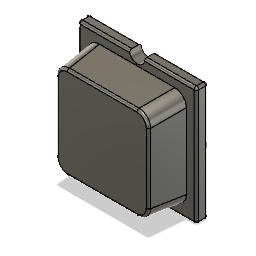
senseCam_Adapter_rev2_enclosure_V2 (Autodesk Fusion 360 archive; units mm, degrees)
design "CA16372_HB-SQ-WWW_Single_Lens"
Autodesk Fusion 360 part; units mm, degrees
sketch "Base 1" plane through (0, 0, 0) normal (0, 0, 1) x (1, 0, 0)
  line L0 (12.5, 12.5) -> (-12.5, 12.5)
  line L1 (-12.5, 12.5) -> (-12.5, -12.5)
  line L2 (-12.5, -12.5) -> (12.5, -12.5)
  line L3 (12.5, -12.5) -> (12.5, 12.5)
  line L4 (12.5, 12.5) -> (-12.5, -12.5) construction
  line L5 (-12.5, 12.5) -> (12.5, -12.5) construction
  line L6 (12.7, 12.7) -> (-12.7, 12.7)
  line L7 (-12.7, 12.7) -> (-12.7, -12.7)
  line L8 (-12.7, -12.7) -> (12.7, -12.7)
  line L9 (12.7, -12.7) -> (12.7, 12.7)
  line L10 (12.7, 12.7) -> (-12.7, -12.7) construction
  line L11 (-12.7, 12.7) -> (12.7, -12.7) construction
  circle A0 centre (0, 12.5) radius 1.6
  circle A1 centre (0, -12.5) radius 1.6
  dimension "d1" = 25
  dimension "d2" = 25
  dimension "d3" = 25.4
  dimension "d4" = 25.4
  dimension "d5" = 3.2
  dimension "d6" = 3.2
  constraint perpendicular L0 L1
  constraint parallel L0 L2
  constraint parallel L1 L3
  constraint horizontal L0
  constraint coincident L4 origin
  constraint coincident L5 origin
  constraint perpendicular L6 L7
  constraint parallel L6 L8
  constraint parallel L7 L9
  constraint horizontal L6
  constraint coincident L10 origin
  constraint coincident L11 origin
  constraint midpoint L0 A0.centre
  constraint midpoint L2 A1.centre
  measures "d1" distance of L0.end L1.end
  measures "d2" distance of L1.end L2.end
  measures "d3" distance of L7.end L8.end
  measures "d4" distance of L6.end L7.end
  measures "d5" diameter of A0
  measures "d6" diameter of A1
extrude "Extrude1" add sketch "Base 1" along normal blind 2.49 contours L0 L1 L2 L3 A0 A1 | L0 L2 L3 L6 L8 L9 A0 A1 | L0 L1 L2 L6 L7 L8 A0 A1
sketch "Lens 1" plane through (0, 0, 2.49) normal (0, 0, 1) x (1, 0, 0)
  line L0 (12.7, -12.7) -> (12.7, 12.7)
  line L1 (12.7, 12.7) -> (1.5875, 12.7)
  arc A0 (-1.5875, 12.7) -> (1.5875, 12.7) centre (0, 12.5) ccw
  line L2 (-1.5875, 12.7) -> (-12.7, 12.7)
  line L3 (-12.7, 12.7) -> (-12.7, -12.7)
  line L4 (-12.7, -12.7) -> (-1.5875, -12.7)
  arc A1 (1.5875, -12.7) -> (-1.5875, -12.7) centre (0, -12.5) ccw
  line L5 (1.5875, -12.7) -> (12.7, -12.7)
  line L6 (10.76, 10.76) -> (-10.76, 10.76)
  line L7 (-10.76, 10.76) -> (-10.76, -10.76)
  line L8 (-10.76, -10.76) -> (10.76, -10.76)
  line L9 (10.76, -10.76) -> (10.76, 10.76)
  line L10 (10.76, 10.76) -> (-10.76, -10.76) construction
  line L11 (-10.76, 10.76) -> (10.76, -10.76) construction
  dimension "d9" = 21.52
  dimension "d10" = 21.52
  constraint perpendicular L6 L7
  constraint parallel L6 L8
  constraint parallel L7 L9
  constraint horizontal L6
  constraint coincident L10 origin
  constraint coincident L11 origin
  measures "d9" distance of L7.end L8.end
  measures "d10" distance of L6.end L7.end
extrude "Extrude2" add sketch "Lens 1" along normal blind 7.47 contours L6 L7 L8 L9
draft "Draft1" angle 5 neutral plane through (0, 0, 0) pull (0, 0, 1) 4 faces at (10.76, -3.5867, 4.98) (-3.5867, -10.76, 4.98) (3.5867, 10.76, 4.98) (-10.76, 3.5867, 4.98)
sketch "Pegs 1" plane through (0, 0, 0) normal (0, 0, -1) x (-1, 0, 0)
  line L0 (-12.7, 12.7) -> (-12.7, -12.7)
  line L1 (-12.7, -12.7) -> (-1.5875, -12.7)
  arc A0 (1.5875, -12.7) -> (-1.5875, -12.7) centre (0, -12.5) ccw
  line L2 (1.5875, -12.7) -> (12.7, -12.7)
  line L3 (12.7, -12.7) -> (12.7, 12.7)
  line L4 (12.7, 12.7) -> (1.5875, 12.7)
  arc A1 (-1.5875, 12.7) -> (1.5875, 12.7) centre (0, 12.5) ccw
  line L5 (-1.5875, 12.7) -> (-12.7, 12.7)
  line L6 (10.77, 10.77) -> (-10.77, 10.77)
  line L7 (-10.77, 10.77) -> (-10.77, -10.77)
  line L8 (-10.77, -10.77) -> (10.77, -10.77)
  line L9 (10.77, -10.77) -> (10.77, 10.77)
  line L10 (10.77, 10.77) -> (-10.77, -10.77) construction
  line L11 (-10.77, 10.77) -> (10.77, -10.77) construction
  circle A2 centre (-10.77, 0) radius 1
  circle A3 centre (10.77, 0) radius 1
  line L12 (10.52, -10.52) -> (10.52, 10.52)
  line L13 (10.52, 10.52) -> (-10.52, 10.52)
  line L14 (-10.52, 10.52) -> (-10.52, -10.52)
  line L15 (-10.52, -10.52) -> (10.52, -10.52)
  dimension "d15" = 21.54
  dimension "d16" = 21.54
  dimension "d17" = 2
  dimension "d18" = 2
  dimension "d19" = -0.25
  constraint perpendicular L6 L7
  constraint parallel L6 L8
  constraint parallel L7 L9
  constraint horizontal L6
  constraint coincident L10 origin
  constraint coincident L11 origin
  constraint midpoint L7 A2.centre
  constraint midpoint L9 A3.centre
  measures "d15" distance of L7.end L8.end
  measures "d16" distance of L6.end L7.end
  measures "d17" diameter of A2
  measures "d18" diameter of A3
extrude "Extrude3" add sketch "Pegs 1" along normal blind 1.1 contours L9 A3 | L9 A3 L12 | L7 A2 L14 | L7 A2
fillet "Fillet1" radius 0.5 18 edges at (11.77, 0, -1.1) (-11.77, 0, -1.1) (-12.7, -12.7, 1.245) (12.7, -12.7, 1.245) (12.7, 12.7, 1.245) (-12.7, 12.7, 1.245) (-7.1437, -12.7, 2.49) (7.1437, -12.7, 2.49) (7.1437, -12.7, 0) (-7.1437, -12.7, 0) (-12.7, 0, 0) (-12.7, 0, 2.49) (7.1437, 12.7, 2.49) (12.7, 0, 2.49) (12.7, 0, 0) (-7.1437, 12.7, 2.49) (-7.1437, 12.7, 0) (7.1437, 12.7, 0)
fillet "Fillet2" radius 2.5 4 edges at (10.2154, 10.2154, 6.225) (-10.2154, 10.2154, 6.225) (-10.2154, -10.2154, 6.225) (10.2154, -10.2154, 6.225)
fillet "Fillet3" radius 0.5 8 edges at (-9.1603, 9.1603, 9.96) (-9.8886, 0, 9.96) (-9.1603, -9.1603, 9.96) (0, -9.8886, 9.96) (9.1603, -9.1603, 9.96) (9.8886, 0, 9.96) (9.1603, 9.1603, 9.96) (0, 9.8886, 9.96)
equation "d7 = ( 9.96 / 4 ) * 1 mm"
equation "d11 = ( ( 9.96 / 4 ) * 3 ) * 1 mm"
named bodies: "90deg Single Lens"
